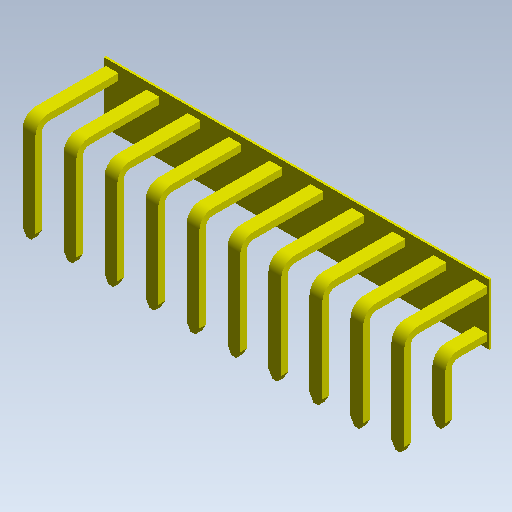
# Autodesk Inventor part: P2SSW-110-02-T-D-RA
Saved by Autodesk Inventor 2021 (Build 250183000, 183)
## iProperties
Part Number: P2SSW-110-02-T-D-RA
Material: Generic
Catalog Web Link: www.cadenas.de
Description: SSW Series Pin-SSW Series - (2,54 mm) .100" Surface Mount Terminal & Through-Hole .025" Square Post Socket
Vendor: SAMTEC
Document SubType Name: Modeling
Designer: partserver
Manufacturer: SAMTEC
Mass: 0.0644753 g
Surface Area: 5.81893 cm^2
Volume: 0.0644753 cm^3
Density: 1 g/cm^3
Appearance: PSOLRGB-255-255-0
Category: PARTsolutions
Company: SAMTEC
PSOL_IDENT_0: {$CADENAS_DATA\23d-libs\samtec\modelling\ssw\parts\ssw_pin.prj},220 {VTYP=3D},{NB=P2SSW-110-02-T-D-R
PSOL_IDENT_1: A},{LINA=P2SSW-110-02-T-D-RA},{NN=SSW Series Pin},{DATE=12.08.2019 09:27:31},{GEOMDATE=07.08.2018 10
PSOL_IDENT_2: :57:54},{VERSION=},{LINEID=10},{WBVAR=POS,LS,PLOPT,ROW,TOPT,POLOPT,LLOPT},{WBNUMERIC=}  {NB=P2SSW-11
PSOL_IDENT_3: 0-02-T-D-RA},{LINA=P2SSW-110-02-T-D-RA},{KT=DUMMY},{PN=SSW-110-02-T-D-RA},{SERIES=SSW},{POS=10},{POS
PSOL_IDENT_4: ATOF=10},{LS=02},{LSALG= '01','-01','02','-02','03','-03','04','-04','06','-06','21','-21','22','-22'
PSOL_IDENT_5: ,'23','-23','24','-24' },{PLOPT=T},{PLOPTALG= 'G','-G - Gold, 20micro\" Au / 50micro\" Ni Min on Con
PSOL_IDENT_6: tact, 3micro\" Au / 50micro\" Ni Min on Tail','S','-S - Selective, 30micro\" Au / 50micro\" Ni Min o
PSOL_IDENT_7: n Contact, Matte Tin Tail','H','-H - Heavy Gold 30micro\" Au / 50micro\" Ni Min on Contact, 3micro\"
PSOL_IDENT_8: Au / 50micro\" Ni Min on Tail' ,'F','-F - Flash Selective, 3micro\" Au / 50micro\" Ni Min on Contac
PSOL_IDENT_9: t, Matte Tin Tail','STL','-STL - Selective, 30micro\" Au / 50micro\" Ni Min on Contact Area, Tin/Lea
PSOL_IDENT_10: d (90/10 +/-5%) Tail','SM','-SM - Selective, 30micro\" Au / 50micro\" Ni Min on Contact, Matte Tin T
PSOL_IDENT_11: ail','FM','-FM - Flash Selective, 3micro\" Au / 50micro\" Ni Min on Contact, Matte Tin Tail','L','-L
PSOL_IDENT_12: - Light Selective, 10micro\" Au / 50micro\" Ni Min on Contact Area, Matte Tin Tail','T','-T - Matte
PSOL_IDENT_13: Tin Contact and Tail','E','-E - 50micro\" Extra Heavy Gold in Contact Area, 3micro\" Gold on Tail','
PSOL_IDENT_14: TM','-TM - Matte Tin Contact and Tail' },{ROW=D},{ROWALG= 'S','-S - Single','D','-D - Double','T','-
PSOL_IDENT_15: T - Triple', 'P','-P - Single Notched','Q','-Q - Triple with only Outer 2 Rows Filled' },{TOPT=RA},{
PSOL_IDENT_16: TOPTALG= '','Straight','RA','-RA - Right Angle' },{TOPTPN=-RA},{POLOPT=},{POLOPTALG= '','Not Selecte
PSOL_IDENT_17: d','001','001','002','002','003','003','004','004','005','005','006','006','007','007','008','008','
PSOL_IDENT_18: 009','009','010','010','011','011','012','012','013','013','014','014','015','015','016','016','017'
PSOL_IDENT_19: ,'017','018','018','019','019','020','020' },{POLOPTMAX=240},{POLOPTMAX2='001','001','002','002','00
PSOL_IDENT_20: 3','003','004','004','005','005','006','006','007','007','008','008','009','009','010','010','011','
PSOL_IDENT_21: 011','012','012','013','013','014','014','015','015','016','016','017','017','018','018','019','019'
PSOL_IDENT_22: ,'020','020'},{POLARIZE='001','001','002','002','003','003','004','004','005','005','006','006','007'
PSOL_IDENT_23: ,'007','008','008','009','009','010','010','011','011','012','012','013','013','014','014','015','01
PSOL_IDENT_24: 5','016','016','017','017','018','018','019','019','020','020','021','021','022','022','023','023','
PSOL_IDENT_25: 024','024','025','025','026','026','027','027','028','028','029','029','030','030','031','031','032'
PSOL_IDENT_26: ,'032','033','033','034','034','035','035','036','036','037','037','038','038','039','039','040','04
PSOL_IDENT_27: 0','041','041','042','042','043','043','044','044','045','045','046','046','047','047','048','048','
PSOL_IDENT_28: 049','049','050','050','051','051','052','052','053','053','054','054','055','055','056','056','057'
PSOL_IDENT_29: ,'057','058','058','059','059','060','060','061','061','062','062','063','063','064','064','065','06
PSOL_IDENT_30: 5','066','066','067','067','068','068','069','069','070','070','071','071','072','072','073','073','
PSOL_IDENT_31: 074','074','075','075','076','076','077','077','078','078','079','079','080','080','081','081','082'
PSOL_IDENT_32: ,'082','083','083','084','084','085','085','086','086','087','087','088','088','089','089','090','09
PSOL_IDENT_33: 0','091','091','092','092','093','093','094','094','095','095','096','096','097','097','098','098','
PSOL_IDENT_34: 099','099','100','100','101','101','102','102','103','103','104','104','105','105','106','106','107'
PSOL_IDENT_35: ,'107','108','108','109','109','110','110','111','111','112','112','113','113','114','114','115','11
PSOL_IDENT_36: 5','116','116','117','117','118','118','119','119','120','120','121','121','122','122','123','123','
PSOL_IDENT_37: 124','124','125','125','126','126','127','127','128','128','129','129','130','130','131','131','132'
PSOL_IDENT_38: ,'132','133','133','134','134','135','135','136','136','137','137','138','138','139','139','140','14
PSOL_IDENT_39: 0','141','141','142','142','143','143','144','144','145','145','146','146','147','147','148','148','
PSOL_IDENT_40: 149','149','150','150'},{POLOPTPN=},{LLOPT=},{LLOPTALG= '','Not Selected','LL','-LL - Locking Lead'
PSOL_IDENT_41: },{LLOPTPN=},{B=0.194},{C=0.100},{R=1.020},{OEN=2}
NB: P2SSW-110-02-T-D-RA
NN: SSW Series Pin
NT: SSW Series - (2,54 mm) .100" Surface Mount Terminal & Through-Hole .025" Square Post Socket
NBSYN: P2$PN.
LINA: P2SSW-110-02-T-D-RA
CATALOG: Samtec
SERIES: SSW
POS: -10
LS: -02
PLOPT: -T - Matte Tin Contact and Tail
ROW: -D - Double
TOPT: -RA - Right Angle
POLOPT: Not Selected
LLOPT: Not Selected
SUPPLIER: SAMTEC
ARTICLENO: P2SSW-110-02-T-D-RA
BOMINFO: P2SSW-110-02-T-D-RA
CREATOR: CADENAS GmbH
Title: P2SSW-110-02-T-D-RA
Author: Cadenas PARTsolutions
Comments: SSW Series - (2,54 mm) .100" Surface Mount Terminal & Through-Hole .025" Square Post Socket
Autodesk Inventor part; units mm, degrees
sketch "Sketch_13" plane through (0, 2.6162, 0) normal (0, 1, 0) x (1, 0, 0)
  line L0 (-11.9507, 1.8796) -> (-11.9507, -1.8796)
  line L1 (-11.9507, -1.8796) -> (11.9507, -1.8796)
  line L2 (11.9507, -1.8796) -> (11.9507, 1.8796)
  line L3 (11.9507, 1.8796) -> (-11.9507, 1.8796)
  constraints: 8 end point
extrude "Extrusion1" add sketch "Sketch_13" along normal blind 0.127
sketch "Sketch_12" plane through (0, 0, 0) normal (1, 0, 0) x (0, 1, 0)
  line L0 (0.4064, 5.0038) -> (0, 5.0038)
  line L1 (0, 5.0038) -> (0, 1.8796)
  arc A0 (0, 1.8796) -> (0.8128, 1.0668) centre (0.8128, 1.8796) ccw
  line L2 (0.8128, 1.0668) -> (2.7432, 1.0668)
  line L3 (2.7432, 1.0668) -> (2.7432, 1.4732)
  line L4 (2.7432, 1.4732) -> (0.8128, 1.4732)
  arc A1 (0.4064, 1.8796) -> (0.8128, 1.4732) centre (0.8128, 1.8796) ccw
  line L5 (0.4064, 1.8796) -> (0.4064, 5.0038)
  constraints: 12 end point, 4 point on circle, 2 centre point
extrude "Extrusion2" add sketch "Sketch_12" along normal mid plane 23.9014
sketch "Sketch_14" plane through (0, 0, 0) normal (1, 0, 0) x (0, 1, 0)
  line L0 (-2.1336, 5.0038) -> (-2.54, 5.0038)
  line L1 (-2.54, 5.0038) -> (-2.54, -0.6604)
  arc A0 (-2.54, -0.6604) -> (-1.7272, -1.4732) centre (-1.7272, -0.6604) ccw
  line L2 (-1.7272, -1.4732) -> (2.7432, -1.4732)
  line L3 (2.7432, -1.4732) -> (2.7432, -1.0668)
  line L4 (2.7432, -1.0668) -> (-1.7272, -1.0668)
  arc A1 (-2.1336, -0.6604) -> (-1.7272, -1.0668) centre (-1.7272, -0.6604) ccw
  line L5 (-2.1336, -0.6604) -> (-2.1336, 5.0038)
  constraints: 12 end point, 4 point on circle, 2 centre point
extrude "Extrusion3" add sketch "Sketch_14" along normal mid plane 23.9014
sketch "Sketch_8" plane through (0, 0, 0) normal (0, 0, 1) x (1, 0, 0)
  line L0 (-13.5763, -22.7838) -> (112.6363, -22.7838)
  line L1 (112.6363, -22.7838) -> (112.6363, 2.6162)
  line L2 (112.6363, 2.6162) -> (110.8837, 2.6162)
  line L3 (110.8837, 2.6162) -> (110.8837, -8.89)
  line L4 (110.8837, -8.89) -> (110.0963, -8.89)
  line L5 (110.0963, -8.89) -> (110.0963, 2.6162)
  line L6 (110.0963, 2.6162) -> (108.3437, 2.6162)
  line L7 (108.3437, 2.6162) -> (108.3437, -8.89)
  line L8 (108.3437, -8.89) -> (107.5563, -8.89)
  line L9 (107.5563, -8.89) -> (107.5563, 2.6162)
  line L10 (107.5563, 2.6162) -> (105.8037, 2.6162)
  line L11 (105.8037, 2.6162) -> (105.8037, -8.89)
  line L12 (105.8037, -8.89) -> (105.0163, -8.89)
  line L13 (105.0163, -8.89) -> (105.0163, 2.6162)
  line L14 (105.0163, 2.6162) -> (103.2637, 2.6162)
  line L15 (103.2637, 2.6162) -> (103.2637, -8.89)
  line L16 (103.2637, -8.89) -> (102.4763, -8.89)
  line L17 (102.4763, -8.89) -> (102.4763, 2.6162)
  line L18 (102.4763, 2.6162) -> (100.7237, 2.6162)
  line L19 (100.7237, 2.6162) -> (100.7237, -8.89)
  line L20 (100.7237, -8.89) -> (99.9363, -8.89)
  line L21 (99.9363, -8.89) -> (99.9363, 2.6162)
  line L22 (99.9363, 2.6162) -> (98.1837, 2.6162)
  line L23 (98.1837, 2.6162) -> (98.1837, -8.89)
  line L24 (98.1837, -8.89) -> (97.3963, -8.89)
  line L25 (97.3963, -8.89) -> (97.3963, 2.6162)
  line L26 (97.3963, 2.6162) -> (95.6437, 2.6162)
  line L27 (95.6437, 2.6162) -> (95.6437, -8.89)
  line L28 (95.6437, -8.89) -> (94.8563, -8.89)
  line L29 (94.8563, -8.89) -> (94.8563, 2.6162)
  line L30 (94.8563, 2.6162) -> (93.1037, 2.6162)
  line L31 (93.1037, 2.6162) -> (93.1037, -8.89)
  line L32 (93.1037, -8.89) -> (92.3163, -8.89)
  line L33 (92.3163, -8.89) -> (92.3163, 2.6162)
  line L34 (92.3163, 2.6162) -> (90.5637, 2.6162)
  line L35 (90.5637, 2.6162) -> (90.5637, -8.89)
  line L36 (90.5637, -8.89) -> (89.7763, -8.89)
  line L37 (89.7763, -8.89) -> (89.7763, 2.6162)
  line L38 (89.7763, 2.6162) -> (88.0237, 2.6162)
  line L39 (88.0237, 2.6162) -> (88.0237, -8.89)
  line L40 (88.0237, -8.89) -> (87.2363, -8.89)
  line L41 (87.2363, -8.89) -> (87.2363, 2.6162)
  line L42 (87.2363, 2.6162) -> (85.4837, 2.6162)
  line L43 (85.4837, 2.6162) -> (85.4837, -8.89)
  line L44 (85.4837, -8.89) -> (84.6963, -8.89)
  line L45 (84.6963, -8.89) -> (84.6963, 2.6162)
  line L46 (84.6963, 2.6162) -> (82.9437, 2.6162)
  line L47 (82.9437, 2.6162) -> (82.9437, -8.89)
  line L48 (82.9437, -8.89) -> (82.1563, -8.89)
  line L49 (82.1563, -8.89) -> (82.1563, 2.6162)
  line L50 (82.1563, 2.6162) -> (80.4037, 2.6162)
  line L51 (80.4037, 2.6162) -> (80.4037, -8.89)
  line L52 (80.4037, -8.89) -> (79.6163, -8.89)
  line L53 (79.6163, -8.89) -> (79.6163, 2.6162)
  line L54 (79.6163, 2.6162) -> (77.8637, 2.6162)
  line L55 (77.8637, 2.6162) -> (77.8637, -8.89)
  line L56 (77.8637, -8.89) -> (77.0763, -8.89)
  line L57 (77.0763, -8.89) -> (77.0763, 2.6162)
  line L58 (77.0763, 2.6162) -> (75.3237, 2.6162)
  line L59 (75.3237, 2.6162) -> (75.3237, -8.89)
  line L60 (75.3237, -8.89) -> (74.5363, -8.89)
  line L61 (74.5363, -8.89) -> (74.5363, 2.6162)
  line L62 (74.5363, 2.6162) -> (72.7837, 2.6162)
  line L63 (72.7837, 2.6162) -> (72.7837, -8.89)
  line L64 (72.7837, -8.89) -> (71.9963, -8.89)
  line L65 (71.9963, -8.89) -> (71.9963, 2.6162)
  line L66 (71.9963, 2.6162) -> (70.2437, 2.6162)
  line L67 (70.2437, 2.6162) -> (70.2437, -8.89)
  line L68 (70.2437, -8.89) -> (69.4563, -8.89)
  line L69 (69.4563, -8.89) -> (69.4563, 2.6162)
  line L70 (69.4563, 2.6162) -> (67.7037, 2.6162)
  line L71 (67.7037, 2.6162) -> (67.7037, -8.89)
  line L72 (67.7037, -8.89) -> (66.9163, -8.89)
  line L73 (66.9163, -8.89) -> (66.9163, 2.6162)
  line L74 (66.9163, 2.6162) -> (65.1637, 2.6162)
  line L75 (65.1637, 2.6162) -> (65.1637, -8.89)
  line L76 (65.1637, -8.89) -> (64.3763, -8.89)
  line L77 (64.3763, -8.89) -> (64.3763, 2.6162)
  line L78 (64.3763, 2.6162) -> (62.6237, 2.6162)
  line L79 (62.6237, 2.6162) -> (62.6237, -8.89)
  line L80 (62.6237, -8.89) -> (61.8363, -8.89)
  line L81 (61.8363, -8.89) -> (61.8363, 2.6162)
  line L82 (61.8363, 2.6162) -> (60.0837, 2.6162)
  line L83 (60.0837, 2.6162) -> (60.0837, -8.89)
  line L84 (60.0837, -8.89) -> (59.2963, -8.89)
  line L85 (59.2963, -8.89) -> (59.2963, 2.6162)
  line L86 (59.2963, 2.6162) -> (57.5437, 2.6162)
  line L87 (57.5437, 2.6162) -> (57.5437, -8.89)
  line L88 (57.5437, -8.89) -> (56.7563, -8.89)
  line L89 (56.7563, -8.89) -> (56.7563, 2.6162)
  line L90 (56.7563, 2.6162) -> (55.0037, 2.6162)
  line L91 (55.0037, 2.6162) -> (55.0037, -8.89)
  line L92 (55.0037, -8.89) -> (54.2163, -8.89)
  line L93 (54.2163, -8.89) -> (54.2163, 2.6162)
  line L94 (54.2163, 2.6162) -> (52.4637, 2.6162)
  line L95 (52.4637, 2.6162) -> (52.4637, -8.89)
  line L96 (52.4637, -8.89) -> (51.6763, -8.89)
  line L97 (51.6763, -8.89) -> (51.6763, 2.6162)
  line L98 (51.6763, 2.6162) -> (49.9237, 2.6162)
  line L99 (49.9237, 2.6162) -> (49.9237, -8.89)
  line L100 (49.9237, -8.89) -> (49.1363, -8.89)
  line L101 (49.1363, -8.89) -> (49.1363, 2.6162)
  line L102 (49.1363, 2.6162) -> (47.3837, 2.6162)
  line L103 (47.3837, 2.6162) -> (47.3837, -8.89)
  line L104 (47.3837, -8.89) -> (46.5963, -8.89)
  line L105 (46.5963, -8.89) -> (46.5963, 2.6162)
  line L106 (46.5963, 2.6162) -> (44.8437, 2.6162)
  line L107 (44.8437, 2.6162) -> (44.8437, -8.89)
  line L108 (44.8437, -8.89) -> (44.0563, -8.89)
  line L109 (44.0563, -8.89) -> (44.0563, 2.6162)
  line L110 (44.0563, 2.6162) -> (42.3037, 2.6162)
  line L111 (42.3037, 2.6162) -> (42.3037, -8.89)
  line L112 (42.3037, -8.89) -> (41.5163, -8.89)
  line L113 (41.5163, -8.89) -> (41.5163, 2.6162)
  line L114 (41.5163, 2.6162) -> (39.7637, 2.6162)
  line L115 (39.7637, 2.6162) -> (39.7637, -8.89)
  line L116 (39.7637, -8.89) -> (38.9763, -8.89)
  line L117 (38.9763, -8.89) -> (38.9763, 2.6162)
  line L118 (38.9763, 2.6162) -> (37.2237, 2.6162)
  line L119 (37.2237, 2.6162) -> (37.2237, -8.89)
  line L120 (37.2237, -8.89) -> (36.4363, -8.89)
  line L121 (36.4363, -8.89) -> (36.4363, 2.6162)
  line L122 (36.4363, 2.6162) -> (34.6837, 2.6162)
  line L123 (34.6837, 2.6162) -> (34.6837, -8.89)
  line L124 (34.6837, -8.89) -> (33.8963, -8.89)
  line L125 (33.8963, -8.89) -> (33.8963, 2.6162)
  line L126 (33.8963, 2.6162) -> (32.1437, 2.6162)
  line L127 (32.1437, 2.6162) -> (32.1437, -8.89)
  line L128 (32.1437, -8.89) -> (31.3563, -8.89)
  line L129 (31.3563, -8.89) -> (31.3563, 2.6162)
  line L130 (31.3563, 2.6162) -> (29.6037, 2.6162)
  line L131 (29.6037, 2.6162) -> (29.6037, -8.89)
  line L132 (29.6037, -8.89) -> (28.8163, -8.89)
  line L133 (28.8163, -8.89) -> (28.8163, 2.6162)
  line L134 (28.8163, 2.6162) -> (27.0637, 2.6162)
  line L135 (27.0637, 2.6162) -> (27.0637, -8.89)
  line L136 (27.0637, -8.89) -> (26.2763, -8.89)
  line L137 (26.2763, -8.89) -> (26.2763, 2.6162)
  line L138 (26.2763, 2.6162) -> (24.5237, 2.6162)
  line L139 (24.5237, 2.6162) -> (24.5237, -8.89)
  line L140 (24.5237, -8.89) -> (23.7363, -8.89)
  line L141 (23.7363, -8.89) -> (23.7363, 2.6162)
  line L142 (23.7363, 2.6162) -> (21.9837, 2.6162)
  line L143 (21.9837, 2.6162) -> (21.9837, -8.89)
  line L144 (21.9837, -8.89) -> (21.1963, -8.89)
  line L145 (21.1963, -8.89) -> (21.1963, 2.6162)
  line L146 (21.1963, 2.6162) -> (19.4437, 2.6162)
  line L147 (19.4437, 2.6162) -> (19.4437, -8.89)
  line L148 (19.4437, -8.89) -> (18.6563, -8.89)
  line L149 (18.6563, -8.89) -> (18.6563, 2.6162)
  line L150 (18.6563, 2.6162) -> (16.9037, 2.6162)
  line L151 (16.9037, 2.6162) -> (16.9037, -8.89)
  line L152 (16.9037, -8.89) -> (16.1163, -8.89)
  line L153 (16.1163, -8.89) -> (16.1163, 2.6162)
  line L154 (16.1163, 2.6162) -> (14.3637, 2.6162)
  line L155 (14.3637, 2.6162) -> (14.3637, -8.89)
  line L156 (14.3637, -8.89) -> (13.5763, -8.89)
  line L157 (13.5763, -8.89) -> (13.5763, 2.6162)
  line L158 (13.5763, 2.6162) -> (11.8237, 2.6162)
  line L159 (11.8237, 2.6162) -> (11.8237, -8.89)
  line L160 (11.8237, -8.89) -> (11.0363, -8.89)
  line L161 (11.0363, -8.89) -> (11.0363, 2.6162)
  line L162 (11.0363, 2.6162) -> (9.2837, 2.6162)
  line L163 (9.2837, 2.6162) -> (9.2837, -8.89)
  line L164 (9.2837, -8.89) -> (8.4963, -8.89)
  line L165 (8.4963, -8.89) -> (8.4963, 2.6162)
  line L166 (8.4963, 2.6162) -> (6.7437, 2.6162)
  line L167 (6.7437, 2.6162) -> (6.7437, -8.89)
  line L168 (6.7437, -8.89) -> (5.9563, -8.89)
  line L169 (5.9563, -8.89) -> (5.9563, 2.6162)
  line L170 (5.9563, 2.6162) -> (4.2037, 2.6162)
  line L171 (4.2037, 2.6162) -> (4.2037, -8.89)
  line L172 (4.2037, -8.89) -> (3.4163, -8.89)
  line L173 (3.4163, -8.89) -> (3.4163, 2.6162)
  line L174 (3.4163, 2.6162) -> (1.6637, 2.6162)
  line L175 (1.6637, 2.6162) -> (1.6637, -8.89)
  line L176 (1.6637, -8.89) -> (0.8763, -8.89)
  line L177 (0.8763, -8.89) -> (0.8763, 2.6162)
  line L178 (0.8763, 2.6162) -> (-0.8763, 2.6162)
  line L179 (-0.8763, 2.6162) -> (-0.8763, -8.89)
  line L180 (-0.8763, -8.89) -> (-1.6637, -8.89)
  line L181 (-1.6637, -8.89) -> (-1.6637, 2.6162)
  line L182 (-1.6637, 2.6162) -> (-3.4163, 2.6162)
  line L183 (-3.4163, 2.6162) -> (-3.4163, -8.89)
  line L184 (-3.4163, -8.89) -> (-4.2037, -8.89)
  line L185 (-4.2037, -8.89) -> (-4.2037, 2.6162)
  line L186 (-4.2037, 2.6162) -> (-5.9563, 2.6162)
  line L187 (-5.9563, 2.6162) -> (-5.9563, -8.89)
  line L188 (-5.9563, -8.89) -> (-6.7437, -8.89)
  line L189 (-6.7437, -8.89) -> (-6.7437, 2.6162)
  line L190 (-6.7437, 2.6162) -> (-8.4963, 2.6162)
  line L191 (-8.4963, 2.6162) -> (-8.4963, -8.89)
  line L192 (-8.4963, -8.89) -> (-9.2837, -8.89)
  line L193 (-9.2837, -8.89) -> (-9.2837, 2.6162)
  line L194 (-9.2837, 2.6162) -> (-11.0363, 2.6162)
  line L195 (-11.0363, 2.6162) -> (-11.0363, -8.89)
  line L196 (-11.0363, -8.89) -> (-11.8237, -8.89)
  line L197 (-11.8237, -8.89) -> (-11.8237, 2.6162)
  line L198 (-11.8237, 2.6162) -> (-13.5763, 2.6162)
  line L199 (-13.5763, 2.6162) -> (-13.5763, -22.7838)
  constraints: 400 end point
extrude "Extrusion4" cut sketch "Sketch_8" along normal mid plane 50.8
sketch "Sketch_11" plane through (0, 0, 0) normal (0, 1, 0) x (-1, 0, 0)
  line L0 (11.8237, 4.5766) -> (11.8237, 7.5565)
  line L1 (11.8237, 7.5565) -> (-11.8237, 7.5565)
  line L2 (-11.8237, 7.5565) -> (-11.8237, 4.5766)
  line L3 (-11.8237, 4.5766) -> (-11.5697, 5.0165)
  line L4 (-11.5697, 5.0165) -> (-11.2903, 5.0165)
  line L5 (-11.2903, 5.0165) -> (-11.0363, 4.5766)
  line L6 (-11.0363, 4.5766) -> (-11.0363, 5.08)
  line L7 (-11.0363, 5.08) -> (-9.2837, 5.08)
  line L8 (-9.2837, 5.08) -> (-9.2837, 4.5766)
  line L9 (-9.2837, 4.5766) -> (-9.0297, 5.0165)
  line L10 (-9.0297, 5.0165) -> (-8.7503, 5.0165)
  line L11 (-8.7503, 5.0165) -> (-8.4963, 4.5766)
  line L12 (-8.4963, 4.5766) -> (-8.4963, 5.08)
  line L13 (-8.4963, 5.08) -> (-6.7437, 5.08)
  line L14 (-6.7437, 5.08) -> (-6.7437, 4.5766)
  line L15 (-6.7437, 4.5766) -> (-6.4897, 5.0165)
  line L16 (-6.4897, 5.0165) -> (-6.2103, 5.0165)
  line L17 (-6.2103, 5.0165) -> (-5.9563, 4.5766)
  line L18 (-5.9563, 4.5766) -> (-5.9563, 5.08)
  line L19 (-5.9563, 5.08) -> (-4.2037, 5.08)
  line L20 (-4.2037, 5.08) -> (-4.2037, 4.5766)
  line L21 (-4.2037, 4.5766) -> (-3.9497, 5.0165)
  line L22 (-3.9497, 5.0165) -> (-3.6703, 5.0165)
  line L23 (-3.6703, 5.0165) -> (-3.4163, 4.5766)
  line L24 (-3.4163, 4.5766) -> (-3.4163, 5.08)
  line L25 (-3.4163, 5.08) -> (-1.6637, 5.08)
  line L26 (-1.6637, 5.08) -> (-1.6637, 4.5766)
  line L27 (-1.6637, 4.5766) -> (-1.4097, 5.0165)
  line L28 (-1.4097, 5.0165) -> (-1.1303, 5.0165)
  line L29 (-1.1303, 5.0165) -> (-0.8763, 4.5766)
  line L30 (-0.8763, 4.5766) -> (-0.8763, 5.08)
  line L31 (-0.8763, 5.08) -> (0.8763, 5.08)
  line L32 (0.8763, 5.08) -> (0.8763, 4.5766)
  line L33 (0.8763, 4.5766) -> (1.1303, 5.0165)
  line L34 (1.1303, 5.0165) -> (1.4097, 5.0165)
  line L35 (1.4097, 5.0165) -> (1.6637, 4.5766)
  line L36 (1.6637, 4.5766) -> (1.6637, 5.08)
  line L37 (1.6637, 5.08) -> (3.4163, 5.08)
  line L38 (3.4163, 5.08) -> (3.4163, 4.5766)
  line L39 (3.4163, 4.5766) -> (3.6703, 5.0165)
  line L40 (3.6703, 5.0165) -> (3.9497, 5.0165)
  line L41 (3.9497, 5.0165) -> (4.2037, 4.5766)
  line L42 (4.2037, 4.5766) -> (4.2037, 5.08)
  line L43 (4.2037, 5.08) -> (5.9563, 5.08)
  line L44 (5.9563, 5.08) -> (5.9563, 4.5766)
  line L45 (5.9563, 4.5766) -> (6.2103, 5.0165)
  line L46 (6.2103, 5.0165) -> (6.4897, 5.0165)
  line L47 (6.4897, 5.0165) -> (6.7437, 4.5766)
  line L48 (6.7437, 4.5766) -> (6.7437, 5.08)
  line L49 (6.7437, 5.08) -> (8.4963, 5.08)
  line L50 (8.4963, 5.08) -> (8.4963, 4.5766)
  line L51 (8.4963, 4.5766) -> (8.7503, 5.0165)
  line L52 (8.7503, 5.0165) -> (9.0297, 5.0165)
  line L53 (9.0297, 5.0165) -> (9.2837, 4.5766)
  line L54 (9.2837, 4.5766) -> (9.2837, 5.08)
  line L55 (9.2837, 5.08) -> (11.0363, 5.08)
  line L56 (11.0363, 5.08) -> (11.0363, 4.5766)
  line L57 (11.0363, 4.5766) -> (11.2903, 5.0165)
  line L58 (11.2903, 5.0165) -> (11.5697, 5.0165)
  line L59 (11.5697, 5.0165) -> (11.8237, 4.5766)
  constraints: 120 end point
extrude "Extrusion5" cut sketch "Sketch_11" along normal mid plane 50.8
ref_plane "pin_XY" through (0, 1.7272, 0) normal (0, -1, 0) x (1, 0, 0)
ref_plane "pin_YZ" through (0, 1.7272, 0) normal (1, 0, 0) x (0, 0, 1)
ref_plane "pin_ZX" through (0, 1.7272, 0) normal (0, 0, 1) x (0, -1, 0)
body "Solid1"
